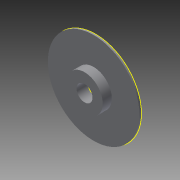
# Autodesk Inventor part: BigPositionDisk
Saved by Autodesk Inventor 2015 (Build 190159000, 159)
## iProperties
Created: 2017-01-31
Part Number: BigPositionDisk
Material: Generic
Document SubType Name: Modeling
Designer: Ernest
Density: 1 g/cm^3
Appearance: Default
Author: Ernest
Autodesk Inventor part; units mm, degrees
ref_plane "YZ Plane" through (0, 0, 0) normal (1, 0, 0) x (0, 1, 0)
ref_plane "XZ Plane" through (0, 0, 0) normal (0, 1, 0) x (-1, 0, 0)
ref_plane "XY Plane" through (0, 0, 0) normal (0, 0, 1) x (1, 0, 0)
sketch "Sketch1" plane through (0, 0, 0) normal (0, 1, 0) x (-1, 0, 0)
  circle A0 centre (0, 0) radius 25.2
  line L0 (0, 0) -> (25.2, 0)
  circle A1 centre (0, 0) radius 4.4
  dimension "d1" = 50.4
  dimension "d6" = 8.8
  constraints: 2 end point, 1 centre point, 1 horizontal, 1 horizontal alignment, 2 other
  measures "d6" diameter of A1
extrude "Extrusion1" add sketch "Sketch1" along normal blind 6
sketch "Sketch2" plane through (0, 0, 0) normal (0, -1, 0) x (1, 0, 0)
  circle A0 centre (0, 0) radius 4.4 projected
  circle A1 centre (0, 0) radius 25.2 projected
  circle A2 centre (0, 0) radius 10
  circle A3 centre (0, 0) radius 25.2
  dimension "d7" = 20
  constraints: 2 centre point, 2 coincident
  measures "d7" diameter of A2
extrude "Extrusion2" cut sketch "Sketch2" against normal blind 5 contours A1
sketch "Sketch4" plane through (0, 6, 0) normal (0, 1, 0) x (1, 0, 0)
  circle A0 centre (0, 0) radius 4.4 projected
  circle A1 centre (0, 0) radius 25.2 projected
  line L0 (0, 0) -> (0, -25.2) construction
  circle A2 centre (0, 0) radius 25.2 projected
  constraints: 2 end point, 2 vertical alignment, 1 vertical, 2 other
body "Solid1"
